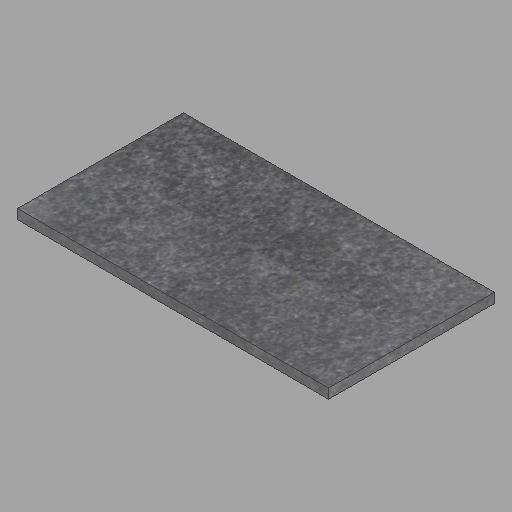
# Autodesk Inventor part: E
Saved by Autodesk Inventor 2023 (Build 270158030, 158C)
## iProperties
RuleStatus: InUse
Created: 2022-05-17
Part Number: E
Material: Granite, Cut, Polished
Document SubType Name: Modeling
Designer: awelt
Mass: 191802 g
Surface Area: 30490.3 cm^2
Volume: 71037.9 cm^3
Density: 2.7 g/cm^3
Appearance: Kasota SN sapphire
AfterDocSave0: in3 to ft3 2
in3 to ft3 2: 0.0
TEST: 0.001
Author: awelt
Autodesk Inventor part; units mm, degrees
ref_plane "YZ Plane" through (0, 0, 0) normal (1, 0, 0) x (0, 1, 0)
ref_plane "XZ Plane" through (0, 0, 0) normal (0, 1, 0) x (-1, 0, 0)
ref_plane "XY Plane" through (0, 0, 0) normal (0, 0, 1) x (1, 0, 0)
sketch "Sketch1" plane through (0, 0, 0) normal (0, 1, 0) x (-1, 0, 0)
  line L0 (0, 0) -> (-1619.25, 0)
  line L1 (-1619.25, 0) -> (-1619.25, -863.6)
  line L2 (-1619.25, -863.6) -> (0, -863.6)
  line L3 (0, -863.6) -> (0, 0)
  dimension "d0" = 1619.25
  dimension "d1" = 863.6
  constraints: 8 end point, 2 parallel, 1 horizontal, 1 perpendicular
  measures "d0" distance of L2.end L1.end
  measures "d1" distance of L1.end L0.end
extrude "Extrusion1" add sketch "Sketch1" along normal blind 50.8
body "Solid1"
